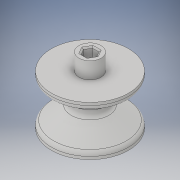
# Autodesk Inventor part: spoolV02
Saved by Autodesk Inventor 2019.3 (Build 233278000, 278)
## iProperties
Created: 2019-02-25
Part Number: spoolV02
Material: Generic
Document SubType Name: Modeling
Designer: steele
Density: 1 g/cm^3
Appearance: Default
Author: steele
Autodesk Inventor part; units mm, degrees
ref_plane "YZ Plane" through (0, 0, 0) normal (1, 0, 0) x (0, 1, 0)
ref_plane "XZ Plane" through (0, 0, 0) normal (0, 1, 0) x (-1, 0, 0)
ref_plane "XY Plane" through (0, 0, 0) normal (0, 0, 1) x (1, 0, 0)
sketch "Sketch1" plane through (0, 0, 0) normal (1, 0, 0) x (0, 1, 0)
  line L0 (0, 0) -> (0, -44.45)
  line L1 (0, 0) -> (57.15, 0)
  line L2 (0, -44.45) -> (6.35, -44.45)
  line L3 (6.35, -44.45) -> (23.495, -21.59)
  line L4 (57.15, 0) -> (76.2, 0)
  line L5 (76.2, 0) -> (76.2, -12.7)
  line L6 (76.2, -12.7) -> (57.15, -12.7)
  line L7 (57.15, -12.7) -> (57.15, -44.45)
  line L8 (57.15, -44.45) -> (50.8, -44.45)
  line L9 (50.8, -44.45) -> (33.655, -21.59)
  arc A0 (33.655, -21.59) -> (23.495, -21.59) centre (28.575, -25.4) ccw
  point P0 (28.575, -14.8167)
  dimension "d36" = 44.45
  dimension "d37" = 57.15
  dimension "d38" = 6.35
  dimension "d40" = 28.575
  dimension "d41" = 19.05
  dimension "d42" = 12.7
  dimension "d43" = 44.45
  dimension "d44" = 57.15
  dimension "d48" = 6.35
  dimension "d53" = 19.05
  constraints: 20 end point, 4 horizontal, 3 perpendicular, 2 point on circle, 2 point on line, 2 tangent, 1 centre point, 1 collinear, 1 vertical
  measures "d36" distance of L0.start L0.end
  measures "d37" distance of L0.start L1.end
  measures "d38" distance of L0.end L2.end
  measures "d40" distance from line of L0 point (28.575, -14.817)
  measures "d41" distance of L1.end L4.end
  measures "d42" distance of L4.end L5.end
  measures "d43" distance from line of L7.end L4
  measures "d44" distance between parallel lines of L7 L0
  measures "d48" radius of A0
  measures "d53" distance edge to line of A0 L1
revolve "Revolution1" add sketch "Sketch1" angle 360 about axis through (0, 0, 0) along (0, 1, 0)
sketch "Sketch6" plane through (0, 76.2, 0) normal (0, 1, 0) x (1, 0, 0)
  line L0 (7.6623, 0) -> (3.8312, -6.6357)
  line L1 (3.8312, -6.6357) -> (-3.8312, -6.6357)
  line L2 (-3.8312, -6.6357) -> (-7.6623, 0)
  line L3 (-7.6623, 0) -> (-3.8312, 6.6357)
  line L4 (-3.8312, 6.6357) -> (3.8312, 6.6358)
  line L5 (3.8312, 6.6358) -> (7.6623, 0)
  point P0 (0, 0)
  point P1 (0, 0)
  dimension "d45" = 13.2715
  constraints: 12 end point, 1 coincident, 1 horizontal, 13 other
  measures "d45" distance between parallel lines of L1 L4
extrude "Extrusion5" cut sketch "Sketch6" against normal through all
chamfer "Chamfer4" distance 1.5875 angle 45 12 edges at (5.7467, 76.2, 3.3179) (5.7467, 76.2, -3.3179) (0, 76.2, -6.6358) (-5.7467, 76.2, -3.3179) (-5.7467, 76.2, 3.3179) (0, 76.2, 6.6357) (-5.7467, 0, -3.3179) (0, 0, -6.6358) (5.7467, 0, -3.3179) (5.7467, 0, 3.3179) (0, 0, 6.6357) (-5.7467, 0, 3.3179)
fillet "Fillet1" radius 6.35 2 edges at (0, 50.8, 44.45) (0, 6.35, 44.45)
equation "\"d36\" = spoolExteriorRadius"
equation "\"d37\" = spoolHeight"
equation "\"d38\" = supportChannels"
equation "\"d40\" = halfSpoolHeight"
equation "\"d41\" = spacerHeight"
equation "\"d43\" = spoolExteriorRadius"
equation "\"d44\" = spoolHeight"
equation "\"d53\" = spoolInteriroRadius"
equation "\"d45\" = hexDiameter"
equation "\"d49\" = hexHoleChamfer"
equation "\"holeForString\" = stringDiameter + clearanceForString"
equation "\"stringDiameter\" = 3"
equation "\"clearanceForString\" = 0.5"
equation "\"spoolHeight\" = 57.15"
equation "\"hexShaftDiameter\" = 12.7"
equation "\"clearanceForHexShaft\" = 0.5715"
equation "\"hexDiameter\" = hexShaftDiameter + clearanceForHexShaft"
equation "\"supportChannels\" = 6.35"
equation "\"spoolInteriorDiameter\" = 38.1"
equation "\"spoolInteriroRadius\" = 0.5 * spoolInteriorDiameter"
equation "\"spoolExteriorDiameter\" = 88.9"
equation "\"spoolExteriorRadius\" = 0.5 * spoolExteriorDiameter"
equation "\"spoolFiletRadius\" = 0.5 * supportChannels"
equation "\"holeCenter\" = 0.25 * spoolHeight - 0.75 * supportChannels"
equation "\"hexHoleChamfer\" = 1.5875"
equation "\"stringHoleCenterFromHexShaft\" = 0.5 * hexDiameter + 0.5 * holeForString"
equation "\"textCircleDiameter\" = 0.75 * spoolExteriorDiameter"
equation "\"textHeight\" = 6.096"
equation "\"textDepth\" = 1.27"
equation "\"stringHoleChamfer\" = 1.5875"
equation "\"halfSpoolHeight\" = 0.5 * spoolHeight"
equation "\"spoolTotalHeight\" = 76.2"
equation "\"spacerHeight\" = spoolTotalHeight - spoolHeight"
body "Solid1"
